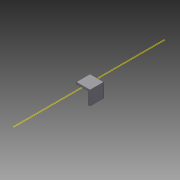
# Autodesk Inventor part: staffa_estrusore
Saved by Autodesk Inventor 2014 SP1 (Build 180222100, 222)
## iProperties
Created: 2015-04-15
Part Number: staffa_estrusore
Material: Generic
Document SubType Name: Modeling
Designer: Giorgio Nuzzo
Density: 1 g/cm^3
Appearance: Default
Author: Giorgio Nuzzo
Autodesk Inventor part; units mm, degrees
ref_plane "YZ Plane" through (0, 0, 0) normal (1, 0, 0) x (0, 1, 0)
ref_plane "XZ Plane" through (0, 0, 0) normal (0, 1, 0) x (-1, 0, 0)
ref_plane "XY Plane" through (0, 0, 0) normal (0, 0, 1) x (1, 0, 0)
ref_plane "Work Plane1" through (56.75, -190.847, 276.8847) normal (0, 0, 1) x (0, 1, 0)
sketch "Sketch1" plane through (56.75, -190.847, 276.8847) normal (0, 0, 1) x (0, 1, 0)
  line L0 (0, 16) -> (395, 16) construction
  line L1 (0, 0) -> (395, 0) construction
  line L2 (177.5, 16) -> (217.5, 16)
  line L3 (217.5, 16) -> (217.5, -24)
  line L4 (217.5, -24) -> (177.5, -24)
  line L5 (177.5, -24) -> (177.5, 16)
  line L6 (197.5, 16) -> (197.5, -37.288) construction
  point P0 (190.847, 56.75)
  dimension "d0" = 40
  dimension "d1" = 40
  constraints: 10 end point, 3 parallel, 2 midpoint, 1 horizontal, 1 perpendicular, 1 other
  measures "d0" distance of L2.start L2.end
  measures "d1" distance of L4.end L2.start
extrude "Extrusion1" add sketch "Sketch1" along normal blind 5
sketch "Sketch2" plane through (56.75, -190.847, 276.8847) normal (0, 0, -1) x (-1, 0, 0)
  line L0 (-24, 177.5) -> (16, 177.5) projected
  line L1 (-24, 217.5) -> (-19, 217.5)
  line L2 (-19, 217.5) -> (-19, 177.5)
  line L3 (-19, 177.5) -> (-24, 177.5)
  line L4 (-24, 177.5) -> (-24, 217.5)
  point P0 (56.75, 190.847)
  dimension "d4" = 5
  constraints: 8 end point, 2 parallel, 1 horizontal, 1 perpendicular, 1 point on line
  measures "d4" distance of L2.end L3.end
extrude "Extrusion2" add sketch "Sketch2" along normal blind 35
body "Solid1"
